Autodesk Inventor part; units mm, degrees
(part 3 of 4)
sketch "Sketch8" plane through (0, 0, 0) normal (0, -1, 0) x (1, 0, 0)
  line L0 (70.4026, -76.6897) -> (69.4026, -74.9577) projected
  line L1 (69.4026, -74.9577) -> (70.4026, -73.2256) projected
  line L2 (70.4026, -73.2256) -> (72.4026, -73.2256) projected
  line L3 (72.4026, -73.2256) -> (73.4026, -74.9577) projected
  line L4 (73.4026, -74.9577) -> (72.4026, -76.6897) projected
  line L5 (72.4026, -76.6897) -> (70.4026, -76.6897) projected
  line L6 (60.9385, -76.6897) -> (59.9385, -74.9577) projected
  line L7 (59.9385, -74.9577) -> (60.9385, -73.2256) projected
  line L8 (60.9385, -73.2256) -> (62.9385, -73.2256) projected
  line L9 (62.9385, -73.2256) -> (63.9385, -74.9577) projected
  line L10 (63.9385, -74.9577) -> (62.9385, -76.6897) projected
  line L11 (62.9385, -76.6897) -> (60.9385, -76.6897) projected
  line L12 (51.4744, -76.6897) -> (50.4744, -74.9577) projected
  line L13 (50.4744, -74.9577) -> (51.4744, -73.2256) projected
  line L14 (51.4744, -73.2256) -> (53.4744, -73.2256) projected
  line L15 (53.4744, -73.2256) -> (54.4744, -74.9577) projected
  line L16 (54.4744, -74.9577) -> (53.4744, -76.6897) projected
  line L17 (53.4744, -76.6897) -> (51.4744, -76.6897) projected
  line L18 (42.0103, -76.6897) -> (41.0103, -74.9577) projected
  line L19 (41.0103, -74.9577) -> (42.0103, -73.2256) projected
  line L20 (42.0103, -73.2256) -> (44.0103, -73.2256) projected
  line L21 (44.0103, -73.2256) -> (45.0103, -74.9577) projected
  line L22 (45.0103, -74.9577) -> (44.0103, -76.6897) projected
  line L23 (44.0103, -76.6897) -> (42.0103, -76.6897) projected
  line L24 (32.5462, -76.6897) -> (31.5462, -74.9577) projected
  line L25 (31.5462, -74.9577) -> (32.5462, -73.2256) projected
  line L26 (32.5462, -73.2256) -> (34.5462, -73.2256) projected
  line L27 (34.5462, -73.2256) -> (35.5462, -74.9577) projected
  line L28 (35.5462, -74.9577) -> (34.5462, -76.6897) projected
  line L29 (34.5462, -76.6897) -> (32.5462, -76.6897) projected
  line L30 (23.0821, -76.6897) -> (22.0821, -74.9577) projected
  line L31 (22.0821, -74.9577) -> (23.0821, -73.2256) projected
  line L32 (23.0821, -73.2256) -> (25.0821, -73.2256) projected
  line L33 (25.0821, -73.2256) -> (26.0821, -74.9577) projected
  line L34 (26.0821, -74.9577) -> (25.0821, -76.6897) projected
  line L35 (25.0821, -76.6897) -> (23.0821, -76.6897) projected
  line L36 (75.1346, -73.9577) -> (74.1346, -72.2256) projected
  line L37 (74.1346, -72.2256) -> (75.1346, -70.4936) projected
  line L38 (75.1346, -70.4936) -> (77.1346, -70.4936) projected
  line L39 (77.1346, -70.4936) -> (78.1346, -72.2256) projected
  line L40 (78.1346, -72.2256) -> (77.1346, -73.9577) projected
  line L41 (77.1346, -73.9577) -> (75.1346, -73.9577) projected
  line L42 (70.4026, -71.2256) -> (69.4026, -69.4936) projected
  line L43 (69.4026, -69.4936) -> (70.4026, -67.7615) projected
  line L44 (70.4026, -67.7615) -> (72.4026, -67.7615) projected
  line L45 (72.4026, -67.7615) -> (73.4026, -69.4936) projected
  line L46 (73.4026, -69.4936) -> (72.4026, -71.2256) projected
  line L47 (72.4026, -71.2256) -> (70.4026, -71.2256) projected
  line L48 (65.6705, -73.9577) -> (64.6705, -72.2256) projected
  line L49 (64.6705, -72.2256) -> (65.6705, -70.4936) projected
  line L50 (65.6705, -70.4936) -> (67.6705, -70.4936) projected
  line L51 (67.6705, -70.4936) -> (68.6705, -72.2256) projected
  line L52 (68.6705, -72.2256) -> (67.6705, -73.9577) projected
  line L53 (67.6705, -73.9577) -> (65.6705, -73.9577) projected
  line L54 (60.9385, -71.2256) -> (59.9385, -69.4936) projected
  line L55 (59.9385, -69.4936) -> (60.9385, -67.7615) projected
  line L56 (60.9385, -67.7615) -> (62.9385, -67.7615) projected
  line L57 (62.9385, -67.7615) -> (63.9385, -69.4936) projected
  line L58 (63.9385, -69.4936) -> (62.9385, -71.2256) projected
  line L59 (62.9385, -71.2256) -> (60.9385, -71.2256) projected
  line L60 (56.2064, -73.9577) -> (55.2064, -72.2256) projected
  line L61 (55.2064, -72.2256) -> (56.2064, -70.4936) projected
  line L62 (56.2064, -70.4936) -> (58.2064, -70.4936) projected
  line L63 (58.2064, -70.4936) -> (59.2064, -72.2256) projected
  line L64 (59.2064, -72.2256) -> (58.2064, -73.9577) projected
  line L65 (58.2064, -73.9577) -> (56.2064, -73.9577) projected
  line L66 (51.4744, -71.2256) -> (50.4744, -69.4936) projected
  line L67 (50.4744, -69.4936) -> (51.4744, -67.7615) projected
  line L68 (51.4744, -67.7615) -> (53.4744, -67.7615) projected
  line L69 (53.4744, -67.7615) -> (54.4744, -69.4936) projected
  line L70 (54.4744, -69.4936) -> (53.4744, -71.2256) projected
  line L71 (53.4744, -71.2256) -> (51.4744, -71.2256) projected
  line L72 (46.7423, -73.9577) -> (45.7423, -72.2256) projected
  line L73 (45.7423, -72.2256) -> (46.7423, -70.4936) projected
  line L74 (46.7423, -70.4936) -> (48.7423, -70.4936) projected
  line L75 (48.7423, -70.4936) -> (49.7423, -72.2256) projected
  line L76 (49.7423, -72.2256) -> (48.7423, -73.9577) projected
  line L77 (48.7423, -73.9577) -> (46.7423, -73.9577) projected
  line L78 (42.0103, -71.2256) -> (41.0103, -69.4936) projected
  line L79 (41.0103, -69.4936) -> (42.0103, -67.7615) projected
  line L80 (42.0103, -67.7615) -> (44.0103, -67.7615) projected
  line L81 (44.0103, -67.7615) -> (45.0103, -69.4936) projected
  line L82 (45.0103, -69.4936) -> (44.0103, -71.2256) projected
  line L83 (44.0103, -71.2256) -> (42.0103, -71.2256) projected
  line L84 (37.2782, -73.9577) -> (36.2782, -72.2256) projected
  line L85 (36.2782, -72.2256) -> (37.2782, -70.4936) projected
  line L86 (37.2782, -70.4936) -> (39.2782, -70.4936) projected
  line L87 (39.2782, -70.4936) -> (40.2782, -72.2256) projected
  line L88 (40.2782, -72.2256) -> (39.2782, -73.9577) projected
  line L89 (39.2782, -73.9577) -> (37.2782, -73.9577) projected
  line L90 (32.5462, -71.2256) -> (31.5462, -69.4936) projected
  line L91 (31.5462, -69.4936) -> (32.5462, -67.7615) projected
  line L92 (32.5462, -67.7615) -> (34.5462, -67.7615) projected
  line L93 (34.5462, -67.7615) -> (35.5462, -69.4936) projected
  line L94 (35.5462, -69.4936) -> (34.5462, -71.2256) projected
  line L95 (34.5462, -71.2256) -> (32.5462, -71.2256) projected
  line L96 (27.8141, -73.9577) -> (26.8141, -72.2256) projected
  line L97 (26.8141, -72.2256) -> (27.8141, -70.4936) projected
  line L98 (27.8141, -70.4936) -> (29.8141, -70.4936) projected
  line L99 (29.8141, -70.4936) -> (30.8141, -72.2256) projected
  line L100 (30.8141, -72.2256) -> (29.8141, -73.9577) projected
  line L101 (29.8141, -73.9577) -> (27.8141, -73.9577) projected
  line L102 (23.0821, -71.2256) -> (22.0821, -69.4936) projected
  line L103 (22.0821, -69.4936) -> (23.0821, -67.7615) projected
  line L104 (23.0821, -67.7615) -> (25.0821, -67.7615) projected
  line L105 (25.0821, -67.7615) -> (26.0821, -69.4936) projected
  line L106 (26.0821, -69.4936) -> (25.0821, -71.2256) projected
  line L107 (25.0821, -71.2256) -> (23.0821, -71.2256) projected
  line L108 (75.1346, -68.4936) -> (74.1346, -66.7615) projected
  line L109 (74.1346, -66.7615) -> (75.1346, -65.0295) projected
  line L110 (75.1346, -65.0295) -> (77.1346, -65.0295) projected
  line L111 (77.1346, -65.0295) -> (78.1346, -66.7615) projected
  line L112 (78.1346, -66.7615) -> (77.1346, -68.4936) projected
  line L113 (77.1346, -68.4936) -> (75.1346, -68.4936) projected
  line L114 (70.4026, -65.7615) -> (69.4026, -64.0295) projected
  line L115 (69.4026, -64.0295) -> (70.4026, -62.2974) projected
  line L116 (70.4026, -62.2974) -> (72.4026, -62.2974) projected
  line L117 (72.4026, -62.2974) -> (73.4026, -64.0295) projected
  line L118 (73.4026, -64.0295) -> (72.4026, -65.7615) projected
  line L119 (72.4026, -65.7615) -> (70.4026, -65.7615) projected
  line L120 (65.6705, -68.4936) -> (64.6705, -66.7615) projected
  line L121 (64.6705, -66.7615) -> (65.6705, -65.0295) projected
  line L122 (65.6705, -65.0295) -> (67.6705, -65.0295) projected
  line L123 (67.6705, -65.0295) -> (68.6705, -66.7615) projected
  line L124 (68.6705, -66.7615) -> (67.6705, -68.4936) projected
  line L125 (67.6705, -68.4936) -> (65.6705, -68.4936) projected
  line L126 (60.9385, -65.7615) -> (59.9385, -64.0295) projected
  line L127 (59.9385, -64.0295) -> (60.9385, -62.2974) projected
  line L128 (60.9385, -62.2974) -> (62.9385, -62.2974) projected
  line L129 (62.9385, -62.2974) -> (63.9385, -64.0295) projected
  line L130 (63.9385, -64.0295) -> (62.9385, -65.7615) projected
  line L131 (62.9385, -65.7615) -> (60.9385, -65.7615) projected
  line L132 (56.2064, -68.4936) -> (55.2064, -66.7615) projected
  line L133 (55.2064, -66.7615) -> (56.2064, -65.0295) projected
  line L134 (56.2064, -65.0295) -> (58.2064, -65.0295) projected
  line L135 (58.2064, -65.0295) -> (59.2064, -66.7615) projected
  line L136 (59.2064, -66.7615) -> (58.2064, -68.4936) projected
  line L137 (58.2064, -68.4936) -> (56.2064, -68.4936) projected
  line L138 (51.4744, -65.7615) -> (50.4744, -64.0295) projected
  line L139 (50.4744, -64.0295) -> (51.4744, -62.2974) projected
  line L140 (51.4744, -62.2974) -> (53.4744, -62.2974) projected
  line L141 (53.4744, -62.2974) -> (54.4744, -64.0295) projected
  line L142 (54.4744, -64.0295) -> (53.4744, -65.7615) projected
  line L143 (53.4744, -65.7615) -> (51.4744, -65.7615) projected
  line L144 (46.7423, -68.4936) -> (45.7423, -66.7615) projected
  line L145 (45.7423, -66.7615) -> (46.7423, -65.0295) projected
  line L146 (46.7423, -65.0295) -> (48.7423, -65.0295) projected
  line L147 (48.7423, -65.0295) -> (49.7423, -66.7615) projected
  line L148 (49.7423, -66.7615) -> (48.7423, -68.4936) projected
  line L149 (48.7423, -68.4936) -> (46.7423, -68.4936) projected
  line L150 (42.0103, -65.7615) -> (41.0103, -64.0295) projected
  line L151 (41.0103, -64.0295) -> (42.0103, -62.2974) projected
  line L152 (42.0103, -62.2974) -> (44.0103, -62.2974) projected
  line L153 (44.0103, -62.2974) -> (45.0103, -64.0295) projected
  line L154 (45.0103, -64.0295) -> (44.0103, -65.7615) projected
  line L155 (44.0103, -65.7615) -> (42.0103, -65.7615) projected
  line L156 (37.2782, -68.4936) -> (36.2782, -66.7615) projected
  line L157 (36.2782, -66.7615) -> (37.2782, -65.0295) projected
  line L158 (37.2782, -65.0295) -> (39.2782, -65.0295) projected
  line L159 (39.2782, -65.0295) -> (40.2782, -66.7615) projected
  line L160 (40.2782, -66.7615) -> (39.2782, -68.4936) projected
  line L161 (39.2782, -68.4936) -> (37.2782, -68.4936) projected
  line L162 (32.5462, -65.7615) -> (31.5462, -64.0295) projected
  line L163 (31.5462, -64.0295) -> (32.5462, -62.2974) projected
  line L164 (32.5462, -62.2974) -> (34.5462, -62.2974) projected
  line L165 (34.5462, -62.2974) -> (35.5462, -64.0295) projected
  line L166 (35.5462, -64.0295) -> (34.5462, -65.7615) projected
  line L167 (34.5462, -65.7615) -> (32.5462, -65.7615) projected
  line L168 (27.8141, -68.4936) -> (26.8141, -66.7615) projected
  line L169 (26.8141, -66.7615) -> (27.8141, -65.0295) projected
  line L170 (27.8141, -65.0295) -> (29.8141, -65.0295) projected
  line L171 (29.8141, -65.0295) -> (30.8141, -66.7615) projected
  line L172 (30.8141, -66.7615) -> (29.8141, -68.4936) projected
  line L173 (29.8141, -68.4936) -> (27.8141, -68.4936) projected
  line L174 (23.0821, -65.7615) -> (22.0821, -64.0295) projected
  line L175 (22.0821, -64.0295) -> (23.0821, -62.2974) projected
  line L176 (23.0821, -62.2974) -> (25.0821, -62.2974) projected
  line L177 (25.0821, -62.2974) -> (26.0821, -64.0295) projected
  line L178 (26.0821, -64.0295) -> (25.0821, -65.7615) projected
  line L179 (25.0821, -65.7615) -> (23.0821, -65.7615) projected
  line L180 (75.1346, -63.0295) -> (74.1346, -61.2974) projected
  line L181 (74.1346, -61.2974) -> (75.1346, -59.5654) projected
  line L182 (75.1346, -59.5654) -> (77.1346, -59.5654) projected
  line L183 (77.1346, -59.5654) -> (78.1346, -61.2974) projected
  line L184 (78.1346, -61.2974) -> (77.1346, -63.0295) projected
  line L185 (77.1346, -63.0295) -> (75.1346, -63.0295) projected
  line L186 (70.4026, -60.2974) -> (69.4026, -58.5654) projected
  line L187 (69.4026, -58.5654) -> (70.4026, -56.8333) projected
  line L188 (70.4026, -56.8333) -> (72.4026, -56.8333) projected
  line L189 (72.4026, -56.8333) -> (73.4026, -58.5654) projected
  line L190 (73.4026, -58.5654) -> (72.4026, -60.2974) projected
  line L191 (72.4026, -60.2974) -> (70.4026, -60.2974) projected
  line L192 (65.6705, -63.0295) -> (64.6705, -61.2974) projected
  line L193 (64.6705, -61.2974) -> (65.6705, -59.5654) projected
  line L194 (65.6705, -59.5654) -> (67.6705, -59.5654) projected
  line L195 (67.6705, -59.5654) -> (68.6705, -61.2974) projected
  line L196 (68.6705, -61.2974) -> (67.6705, -63.0295) projected
  line L197 (67.6705, -63.0295) -> (65.6705, -63.0295) projected
  line L198 (60.9385, -60.2974) -> (59.9385, -58.5654) projected
  line L199 (59.9385, -58.5654) -> (60.9385, -56.8333) projected
  line L200 (60.9385, -56.8333) -> (62.9385, -56.8333) projected
  line L201 (62.9385, -56.8333) -> (63.9385, -58.5654) projected
  line L202 (63.9385, -58.5654) -> (62.9385, -60.2974) projected
  line L203 (62.9385, -60.2974) -> (60.9385, -60.2974) projected
  line L204 (56.2064, -63.0295) -> (55.2064, -61.2974) projected
  line L205 (55.2064, -61.2974) -> (56.2064, -59.5654) projected
  line L206 (56.2064, -59.5654) -> (58.2064, -59.5654) projected
  line L207 (58.2064, -59.5654) -> (59.2064, -61.2974) projected
  line L208 (59.2064, -61.2974) -> (58.2064, -63.0295) projected
  line L209 (58.2064, -63.0295) -> (56.2064, -63.0295) projected
  line L210 (51.4744, -60.2974) -> (50.4744, -58.5654) projected
  line L211 (50.4744, -58.5654) -> (51.4744, -56.8333) projected
  line L212 (51.4744, -56.8333) -> (53.4744, -56.8333) projected
  line L213 (53.4744, -56.8333) -> (54.4744, -58.5654) projected
  line L214 (54.4744, -58.5654) -> (53.4744, -60.2974) projected
  line L215 (53.4744, -60.2974) -> (51.4744, -60.2974) projected
  line L216 (46.7423, -63.0295) -> (45.7423, -61.2974) projected
  line L217 (45.7423, -61.2974) -> (46.7423, -59.5654) projected
  line L218 (46.7423, -59.5654) -> (48.7423, -59.5654) projected
  line L219 (48.7423, -59.5654) -> (49.7423, -61.2974) projected
  line L220 (49.7423, -61.2974) -> (48.7423, -63.0295) projected
  line L221 (48.7423, -63.0295) -> (46.7423, -63.0295) projected
  line L222 (42.0103, -60.2974) -> (41.0103, -58.5654) projected
  line L223 (41.0103, -58.5654) -> (42.0103, -56.8333) projected
  line L224 (42.0103, -56.8333) -> (44.0103, -56.8333) projected
  line L225 (44.0103, -56.8333) -> (45.0103, -58.5654) projected
  line L226 (45.0103, -58.5654) -> (44.0103, -60.2974) projected
  line L227 (44.0103, -60.2974) -> (42.0103, -60.2974) projected
  line L228 (37.2782, -63.0295) -> (36.2782, -61.2974) projected
  line L229 (36.2782, -61.2974) -> (37.2782, -59.5654) projected
  line L230 (37.2782, -59.5654) -> (39.2782, -59.5654) projected
  line L231 (39.2782, -59.5654) -> (40.2782, -61.2974) projected
  line L232 (40.2782, -61.2974) -> (39.2782, -63.0295) projected
  line L233 (39.2782, -63.0295) -> (37.2782, -63.0295) projected
  line L234 (32.5462, -60.2974) -> (31.5462, -58.5654) projected
  line L235 (31.5462, -58.5654) -> (32.5462, -56.8333) projected
  line L236 (32.5462, -56.8333) -> (34.5462, -56.8333) projected
  line L237 (34.5462, -56.8333) -> (35.5462, -58.5654) projected
  line L238 (35.5462, -58.5654) -> (34.5462, -60.2974) projected
  line L239 (34.5462, -60.2974) -> (32.5462, -60.2974) projected
  line L240 (27.8141, -63.0295) -> (26.8141, -61.2974) projected
  line L241 (26.8141, -61.2974) -> (27.8141, -59.5654) projected
  line L242 (27.8141, -59.5654) -> (29.8141, -59.5654) projected
  line L243 (29.8141, -59.5654) -> (30.8141, -61.2974) projected
  line L244 (30.8141, -61.2974) -> (29.8141, -63.0295) projected
  line L245 (29.8141, -63.0295) -> (27.8141, -63.0295) projected
  line L246 (23.0821, -60.2974) -> (22.0821, -58.5654) projected
  line L247 (22.0821, -58.5654) -> (23.0821, -56.8333) projected
  line L248 (23.0821, -56.8333) -> (25.0821, -56.8333) projected
  line L249 (25.0821, -56.8333) -> (26.0821, -58.5654) projected
  line L250 (26.0821, -58.5654) -> (25.0821, -60.2974) projected
  line L251 (25.0821, -60.2974) -> (23.0821, -60.2974) projected
  line L252 (75.1346, -57.5654) -> (74.1346, -55.8333) projected
  line L253 (74.1346, -55.8333) -> (75.1346, -54.1013) projected
  line L254 (75.1346, -54.1013) -> (77.1346, -54.1013) projected
  line L255 (77.1346, -54.1013) -> (78.1346, -55.8333) projected
  line L256 (78.1346, -55.8333) -> (77.1346, -57.5654) projected
  line L257 (77.1346, -57.5654) -> (75.1346, -57.5654) projected
  line L258 (70.4026, -54.8333) -> (69.4026, -53.1013) projected
  line L259 (69.4026, -53.1013) -> (70.4026, -51.3692) projected
  line L260 (70.4026, -51.3692) -> (72.4026, -51.3692) projected
  line L261 (72.4026, -51.3692) -> (73.4026, -53.1013) projected
  line L262 (73.4026, -53.1013) -> (72.4026, -54.8333) projected
  line L263 (72.4026, -54.8333) -> (70.4026, -54.8333) projected
  line L264 (65.6705, -57.5654) -> (64.6705, -55.8333) projected
  line L265 (64.6705, -55.8333) -> (65.6705, -54.1013) projected
  line L266 (65.6705, -54.1013) -> (67.6705, -54.1013) projected
  line L267 (67.6705, -54.1013) -> (68.6705, -55.8333) projected
  line L268 (68.6705, -55.8333) -> (67.6705, -57.5654) projected
  line L269 (67.6705, -57.5654) -> (65.6705, -57.5654) projected
  line L270 (60.9385, -54.8333) -> (59.9385, -53.1013) projected
  line L271 (59.9385, -53.1013) -> (60.9385, -51.3692) projected
  line L272 (60.9385, -51.3692) -> (62.9385, -51.3692) projected
  line L273 (62.9385, -51.3692) -> (63.9385, -53.1013) projected
  line L274 (63.9385, -53.1013) -> (62.9385, -54.8333) projected
  line L275 (62.9385, -54.8333) -> (60.9385, -54.8333) projected
  line L276 (56.2064, -57.5654) -> (55.2064, -55.8333) projected
  line L277 (55.2064, -55.8333) -> (56.2064, -54.1013) projected
  line L278 (56.2064, -54.1013) -> (58.2064, -54.1013) projected
  line L279 (58.2064, -54.1013) -> (59.2064, -55.8333) projected
  line L280 (59.2064, -55.8333) -> (58.2064, -57.5654) projected
  line L281 (58.2064, -57.5654) -> (56.2064, -57.5654) projected
  line L282 (51.4744, -54.8333) -> (50.4744, -53.1013) projected
  line L283 (50.4744, -53.1013) -> (51.4744, -51.3692) projected
  line L284 (51.4744, -51.3692) -> (53.4744, -51.3692) projected
  line L285 (53.4744, -51.3692) -> (54.4744, -53.1013) projected
  line L286 (54.4744, -53.1013) -> (53.4744, -54.8333) projected
  line L287 (53.4744, -54.8333) -> (51.4744, -54.8333) projected
  line L288 (46.7423, -57.5654) -> (45.7423, -55.8333) projected
  line L289 (45.7423, -55.8333) -> (46.7423, -54.1013) projected
  line L290 (46.7423, -54.1013) -> (48.7423, -54.1013) projected
  line L291 (48.7423, -54.1013) -> (49.7423, -55.8333) projected
  line L292 (49.7423, -55.8333) -> (48.7423, -57.5654) projected
  line L293 (48.7423, -57.5654) -> (46.7423, -57.5654) projected
  line L294 (42.0103, -54.8333) -> (41.0103, -53.1013) projected
  line L295 (41.0103, -53.1013) -> (42.0103, -51.3692) projected
  line L296 (42.0103, -51.3692) -> (44.0103, -51.3692) projected
  line L297 (44.0103, -51.3692) -> (45.0103, -53.1013) projected
  line L298 (45.0103, -53.1013) -> (44.0103, -54.8333) projected
  line L299 (44.0103, -54.8333) -> (42.0103, -54.8333) projected
  line L300 (37.2782, -57.5654) -> (36.2782, -55.8333) projected
  line L301 (36.2782, -55.8333) -> (37.2782, -54.1013) projected
  line L302 (37.2782, -54.1013) -> (39.2782, -54.1013) projected
  line L303 (39.2782, -54.1013) -> (40.2782, -55.8333) projected
  line L304 (40.2782, -55.8333) -> (39.2782, -57.5654) projected
  line L305 (39.2782, -57.5654) -> (37.2782, -57.5654) projected
  line L306 (32.5462, -54.8333) -> (31.5462, -53.1013) projected
  line L307 (31.5462, -53.1013) -> (32.5462, -51.3692) projected
  line L308 (32.5462, -51.3692) -> (34.5462, -51.3692) projected
  line L309 (34.5462, -51.3692) -> (35.5462, -53.1013) projected
  line L310 (35.5462, -53.1013) -> (34.5462, -54.8333) projected
  line L311 (34.5462, -54.8333) -> (32.5462, -54.8333) projected
  line L312 (27.8141, -57.5654) -> (26.8141, -55.8333) projected
  line L313 (26.8141, -55.8333) -> (27.8141, -54.1013) projected
  line L314 (27.8141, -54.1013) -> (29.8141, -54.1013) projected
  line L315 (29.8141, -54.1013) -> (30.8141, -55.8333) projected
  line L316 (30.8141, -55.8333) -> (29.8141, -57.5654) projected
  line L317 (29.8141, -57.5654) -> (27.8141, -57.5654) projected
  line L318 (23.0821, -54.8333) -> (22.0821, -53.1013) projected
  line L319 (22.0821, -53.1013) -> (23.0821, -51.3692) projected
  line L320 (23.0821, -51.3692) -> (25.0821, -51.3692) projected
  line L321 (25.0821, -51.3692) -> (26.0821, -53.1013) projected
  line L322 (26.0821, -53.1013) -> (25.0821, -54.8333) projected
  line L323 (25.0821, -54.8333) -> (23.0821, -54.8333) projected
  line L324 (75.1346, -52.1013) -> (74.1346, -50.3692) projected
  line L325 (74.1346, -50.3692) -> (75.1346, -48.6372) projected
  line L326 (75.1346, -48.6372) -> (77.1346, -48.6372) projected
  line L327 (77.1346, -48.6372) -> (78.1346, -50.3692) projected
  line L328 (78.1346, -50.3692) -> (77.1346, -52.1013) projected
  line L329 (77.1346, -52.1013) -> (75.1346, -52.1013) projected
  line L330 (70.4026, -49.3692) -> (69.4026, -47.6372) projected
  line L331 (69.4026, -47.6372) -> (70.4026, -45.9051) projected
  line L332 (70.4026, -45.9051) -> (72.4026, -45.9051) projected
  line L333 (72.4026, -45.9051) -> (73.4026, -47.6372) projected
  line L334 (73.4026, -47.6372) -> (72.4026, -49.3692) projected
  line L335 (72.4026, -49.3692) -> (70.4026, -49.3692) projected
  line L336 (65.6705, -52.1013) -> (64.6705, -50.3692) projected
  line L337 (64.6705, -50.3692) -> (65.6705, -48.6372) projected
  line L338 (65.6705, -48.6372) -> (67.6705, -48.6372) projected
  line L339 (67.6705, -48.6372) -> (68.6705, -50.3692) projected
  line L340 (68.6705, -50.3692) -> (67.6705, -52.1013) projected
  line L341 (67.6705, -52.1013) -> (65.6705, -52.1013) projected
  line L342 (60.9385, -49.3692) -> (59.9385, -47.6372) projected
  line L343 (59.9385, -47.6372) -> (60.9385, -45.9051) projected
  line L344 (60.9385, -45.9051) -> (62.9385, -45.9051) projected
  line L345 (62.9385, -45.9051) -> (63.9385, -47.6372) projected
  line L346 (63.9385, -47.6372) -> (62.9385, -49.3692) projected
  line L347 (62.9385, -49.3692) -> (60.9385, -49.3692) projected
  line L348 (56.2064, -52.1013) -> (55.2064, -50.3692) projected
  line L349 (55.2064, -50.3692) -> (56.2064, -48.6372) projected
  line L350 (56.2064, -48.6372) -> (58.2064, -48.6372) projected
  line L351 (58.2064, -48.6372) -> (59.2064, -50.3692) projected
  line L352 (59.2064, -50.3692) -> (58.2064, -52.1013) projected
  line L353 (58.2064, -52.1013) -> (56.2064, -52.1013) projected
  line L354 (51.4744, -49.3692) -> (50.4744, -47.6372) projected
  line L355 (50.4744, -47.6372) -> (51.4744, -45.9051) projected
  line L356 (51.4744, -45.9051) -> (53.4744, -45.9051) projected
  line L357 (53.4744, -45.9051) -> (54.4744, -47.6372) projected
  line L358 (54.4744, -47.6372) -> (53.4744, -49.3692) projected
  line L359 (53.4744, -49.3692) -> (51.4744, -49.3692) projected
  line L360 (46.7423, -52.1013) -> (45.7423, -50.3692) projected
  line L361 (45.7423, -50.3692) -> (46.7423, -48.6372) projected
  line L362 (46.7423, -48.6372) -> (48.7423, -48.6372) projected
  line L363 (48.7423, -48.6372) -> (49.7423, -50.3692) projected
  line L364 (49.7423, -50.3692) -> (48.7423, -52.1013) projected
  line L365 (48.7423, -52.1013) -> (46.7423, -52.1013) projected
  line L366 (42.0103, -49.3692) -> (41.0103, -47.6372) projected
  line L367 (41.0103, -47.6372) -> (42.0103, -45.9051) projected
  line L368 (42.0103, -45.9051) -> (44.0103, -45.9051) projected
  line L369 (44.0103, -45.9051) -> (45.0103, -47.6372) projected
  line L370 (45.0103, -47.6372) -> (44.0103, -49.3692) projected
  line L371 (44.0103, -49.3692) -> (42.0103, -49.3692) projected
  line L372 (37.2782, -52.1013) -> (36.2782, -50.3692) projected
  line L373 (36.2782, -50.3692) -> (37.2782, -48.6372) projected
  line L374 (37.2782, -48.6372) -> (39.2782, -48.6372) projected
  line L375 (39.2782, -48.6372) -> (40.2782, -50.3692) projected
  line L376 (40.2782, -50.3692) -> (39.2782, -52.1013) projected
  line L377 (39.2782, -52.1013) -> (37.2782, -52.1013) projected
  line L378 (32.5462, -49.3692) -> (31.5462, -47.6372) projected
  line L379 (31.5462, -47.6372) -> (32.5462, -45.9051) projected
  line L380 (32.5462, -45.9051) -> (34.5462, -45.9051) projected
  line L381 (34.5462, -45.9051) -> (35.5462, -47.6372) projected
  line L382 (35.5462, -47.6372) -> (34.5462, -49.3692) projected
  line L383 (34.5462, -49.3692) -> (32.5462, -49.3692) projected
  line L384 (27.8141, -52.1013) -> (26.8141, -50.3692) projected
  line L385 (26.8141, -50.3692) -> (27.8141, -48.6372) projected
  line L386 (27.8141, -48.6372) -> (29.8141, -48.6372) projected
  line L387 (29.8141, -48.6372) -> (30.8141, -50.3692) projected
  line L388 (30.8141, -50.3692) -> (29.8141, -52.1013) projected
  line L389 (29.8141, -52.1013) -> (27.8141, -52.1013) projected
  line L390 (23.0821, -49.3692) -> (22.0821, -47.6372) projected
  line L391 (22.0821, -47.6372) -> (23.0821, -45.9051) projected
  line L392 (23.0821, -45.9051) -> (25.0821, -45.9051) projected
  line L393 (25.0821, -45.9051) -> (26.0821, -47.6372) projected
  line L394 (26.0821, -47.6372) -> (25.0821, -49.3692) projected
  line L395 (25.0821, -49.3692) -> (23.0821, -49.3692) projected
  line L396 (75.1346, -46.6372) -> (74.1346, -44.9051) projected
  line L397 (74.1346, -44.9051) -> (75.1346, -43.1731) projected
  line L398 (75.1346, -43.1731) -> (77.1346, -43.1731) projected
  line L399 (77.1346, -43.1731) -> (78.1346, -44.9051) projected
  line L400 (78.1346, -44.9051) -> (77.1346, -46.6372) projected
  line L401 (77.1346, -46.6372) -> (75.1346, -46.6372) projected
  line L402 (70.4026, -43.9051) -> (69.4026, -42.1731) projected
  line L403 (69.4026, -42.1731) -> (70.4026, -40.441) projected
  line L404 (70.4026, -40.441) -> (72.4026, -40.441) projected
  line L405 (72.4026, -40.441) -> (73.4026, -42.1731) projected
  line L406 (73.4026, -42.1731) -> (72.4026, -43.9051) projected
  line L407 (72.4026, -43.9051) -> (70.4026, -43.9051) projected
  line L408 (65.6705, -46.6372) -> (64.6705, -44.9051) projected
  line L409 (64.6705, -44.9051) -> (65.6705, -43.1731) projected
  line L410 (65.6705, -43.1731) -> (67.6705, -43.1731) projected
  line L411 (67.6705, -43.1731) -> (68.6705, -44.9051) projected
  line L412 (68.6705, -44.9051) -> (67.6705, -46.6372) projected
  line L413 (67.6705, -46.6372) -> (65.6705, -46.6372) projected
  line L414 (60.9385, -43.9051) -> (59.9385, -42.1731) projected
  line L415 (59.9385, -42.1731) -> (60.9385, -40.441) projected
  line L416 (60.9385, -40.441) -> (62.9385, -40.441) projected
  line L417 (62.9385, -40.441) -> (63.9385, -42.1731) projected
  line L418 (63.9385, -42.1731) -> (62.9385, -43.9051) projected
  line L419 (62.9385, -43.9051) -> (60.9385, -43.9051) projected
  line L420 (56.2064, -46.6372) -> (55.2064, -44.9051) projected
  line L421 (55.2064, -44.9051) -> (56.2064, -43.1731) projected
  line L422 (56.2064, -43.1731) -> (58.2064, -43.1731) projected
  line L423 (58.2064, -43.1731) -> (59.2064, -44.9051) projected
  line L424 (59.2064, -44.9051) -> (58.2064, -46.6372) projected
  line L425 (58.2064, -46.6372) -> (56.2064, -46.6372) projected
  line L426 (51.4744, -43.9051) -> (50.4744, -42.1731) projected
  line L427 (50.4744, -42.1731) -> (51.4744, -40.441) projected
  line L428 (51.4744, -40.441) -> (53.4744, -40.441) projected
  line L429 (53.4744, -40.441) -> (54.4744, -42.1731) projected
  line L430 (54.4744, -42.1731) -> (53.4744, -43.9051) projected
  line L431 (53.4744, -43.9051) -> (51.4744, -43.9051) projected
  line L432 (46.7423, -46.6372) -> (45.7423, -44.9051) projected
  line L433 (45.7423, -44.9051) -> (46.7423, -43.1731) projected
  line L434 (46.7423, -43.1731) -> (48.7423, -43.1731) projected
  line L435 (48.7423, -43.1731) -> (49.7423, -44.9051) projected
  line L436 (49.7423, -44.9051) -> (48.7423, -46.6372) projected
  line L437 (48.7423, -46.6372) -> (46.7423, -46.6372) projected
  line L438 (42.0103, -43.9051) -> (41.0103, -42.1731) projected
  line L439 (41.0103, -42.1731) -> (42.0103, -40.441) projected
  line L440 (42.0103, -40.441) -> (44.0103, -40.441) projected
  line L441 (44.0103, -40.441) -> (45.0103, -42.1731) projected
  line L442 (45.0103, -42.1731) -> (44.0103, -43.9051) projected
  line L443 (44.0103, -43.9051) -> (42.0103, -43.9051) projected
  line L444 (37.2782, -46.6372) -> (36.2782, -44.9051) projected
  line L445 (36.2782, -44.9051) -> (37.2782, -43.1731) projected
  line L446 (37.2782, -43.1731) -> (39.2782, -43.1731) projected
  line L447 (39.2782, -43.1731) -> (40.2782, -44.9051) projected
  line L448 (40.2782, -44.9051) -> (39.2782, -46.6372) projected
  line L449 (39.2782, -46.6372) -> (37.2782, -46.6372) projected
  line L450 (32.5462, -43.9051) -> (31.5462, -42.1731) projected
  line L451 (31.5462, -42.1731) -> (32.5462, -40.441) projected
  line L452 (32.5462, -40.441) -> (34.5462, -40.441) projected
  line L453 (34.5462, -40.441) -> (35.5462, -42.1731) projected
  line L454 (35.5462, -42.1731) -> (34.5462, -43.9051) projected
  line L455 (34.5462, -43.9051) -> (32.5462, -43.9051) projected
  line L456 (27.8141, -46.6372) -> (26.8141, -44.9051) projected
  line L457 (26.8141, -44.9051) -> (27.8141, -43.1731) projected
  line L458 (27.8141, -43.1731) -> (29.8141, -43.1731) projected
  line L459 (29.8141, -43.1731) -> (30.8141, -44.9051) projected
  line L460 (30.8141, -44.9051) -> (29.8141, -46.6372) projected
  line L461 (29.8141, -46.6372) -> (27.8141, -46.6372) projected
  line L462 (23.0821, -43.9051) -> (22.0821, -42.1731) projected
  line L463 (22.0821, -42.1731) -> (23.0821, -40.441) projected
  line L464 (23.0821, -40.441) -> (25.0821, -40.441) projected
  line L465 (25.0821, -40.441) -> (26.0821, -42.1731) projected
  line L466 (26.0821, -42.1731) -> (25.0821, -43.9051) projected
  line L467 (25.0821, -43.9051) -> (23.0821, -43.9051) projected
  line L468 (75.1346, -41.1731) -> (74.1346, -39.441) projected
  line L469 (74.1346, -39.441) -> (75.1346, -37.709) projected
  line L470 (75.1346, -37.709) -> (77.1346, -37.709) projected
  line L471 (77.1346, -37.709) -> (78.1346, -39.441) projected
  line L472 (78.1346, -39.441) -> (77.1346, -41.1731) projected
  line L473 (77.1346, -41.1731) -> (75.1346, -41.1731) projected
  line L474 (70.4026, -38.441) -> (69.4026, -36.709) projected
  line L475 (69.4026, -36.709) -> (70.4026, -34.9769) projected
  line L476 (70.4026, -34.9769) -> (72.4026, -34.9769) projected
  line L477 (72.4026, -34.9769) -> (73.4026, -36.709) projected
  line L478 (73.4026, -36.709) -> (72.4026, -38.441) projected
  line L479 (72.4026, -38.441) -> (70.4026, -38.441) projected
  line L480 (65.6705, -41.1731) -> (64.6705, -39.441) projected
  line L481 (64.6705, -39.441) -> (65.6705, -37.709) projected
  line L482 (65.6705, -37.709) -> (67.6705, -37.709) projected
  line L483 (67.6705, -37.709) -> (68.6705, -39.441) projected
  line L484 (68.6705, -39.441) -> (67.6705, -41.1731) projected
  line L485 (67.6705, -41.1731) -> (65.6705, -41.1731) projected
  line L486 (60.9385, -38.441) -> (59.9385, -36.709) projected
  line L487 (59.9385, -36.709) -> (60.9385, -34.9769) projected
  line L488 (60.9385, -34.9769) -> (62.9385, -34.9769) projected
  line L489 (62.9385, -34.9769) -> (63.9385, -36.709) projected
  line L490 (63.9385, -36.709) -> (62.9385, -38.441) projected
  line L491 (62.9385, -38.441) -> (60.9385, -38.441) projected
  line L492 (56.2064, -41.1731) -> (55.2064, -39.441) projected
  line L493 (55.2064, -39.441) -> (56.2064, -37.709) projected
  line L494 (56.2064, -37.709) -> (58.2064, -37.709) projected
  line L495 (58.2064, -37.709) -> (59.2064, -39.441) projected
  line L496 (59.2064, -39.441) -> (58.2064, -41.1731) projected
  line L497 (58.2064, -41.1731) -> (56.2064, -41.1731) projected
  line L498 (51.4744, -38.441) -> (50.4744, -36.709) projected
  line L499 (50.4744, -36.709) -> (51.4744, -34.9769) projected
  line L500 (51.4744, -34.9769) -> (53.4744, -34.9769) projected
  line L501 (53.4744, -34.9769) -> (54.4744, -36.709) projected
  line L502 (54.4744, -36.709) -> (53.4744, -38.441) projected
  line L503 (53.4744, -38.441) -> (51.4744, -38.441) projected
  line L504 (46.7423, -41.1731) -> (45.7423, -39.441) projected
  line L505 (45.7423, -39.441) -> (46.7423, -37.709) projected
  line L506 (46.7423, -37.709) -> (48.7423, -37.709) projected
  line L507 (48.7423, -37.709) -> (49.7423, -39.441) projected
  line L508 (49.7423, -39.441) -> (48.7423, -41.1731) projected
  line L509 (48.7423, -41.1731) -> (46.7423, -41.1731) projected
  line L510 (42.0103, -38.441) -> (41.0103, -36.709) projected
  line L511 (41.0103, -36.709) -> (42.0103, -34.9769) projected
  line L512 (42.0103, -34.9769) -> (44.0103, -34.9769) projected
  line L513 (44.0103, -34.9769) -> (45.0103, -36.709) projected
  line L514 (45.0103, -36.709) -> (44.0103, -38.441) projected
  line L515 (44.0103, -38.441) -> (42.0103, -38.441) projected
  line L516 (37.2782, -41.1731) -> (36.2782, -39.441) projected
  line L517 (36.2782, -39.441) -> (37.2782, -37.709) projected
  line L518 (37.2782, -37.709) -> (39.2782, -37.709) projected
  line L519 (39.2782, -37.709) -> (40.2782, -39.441) projected
  line L520 (40.2782, -39.441) -> (39.2782, -41.1731) projected
  line L521 (39.2782, -41.1731) -> (37.2782, -41.1731) projected
  line L522 (32.5462, -38.441) -> (31.5462, -36.709) projected
  line L523 (31.5462, -36.709) -> (32.5462, -34.9769) projected
  line L524 (32.5462, -34.9769) -> (34.5462, -34.9769) projected
  line L525 (34.5462, -34.9769) -> (35.5462, -36.709) projected
  line L526 (35.5462, -36.709) -> (34.5462, -38.441) projected
  line L527 (34.5462, -38.441) -> (32.5462, -38.441) projected
  line L528 (27.8141, -41.1731) -> (26.8141, -39.441) projected
  line L529 (26.8141, -39.441) -> (27.8141, -37.709) projected
  line L530 (27.8141, -37.709) -> (29.8141, -37.709) projected
  line L531 (29.8141, -37.709) -> (30.8141, -39.441) projected
  line L532 (30.8141, -39.441) -> (29.8141, -41.1731) projected
  line L533 (29.8141, -41.1731) -> (27.8141, -41.1731) projected
  line L534 (23.0821, -38.441) -> (22.0821, -36.709) projected
  line L535 (22.0821, -36.709) -> (23.0821, -34.9769) projected
  line L536 (23.0821, -34.9769) -> (25.0821, -34.9769) projected
  line L537 (25.0821, -34.9769) -> (26.0821, -36.709) projected
  line L538 (26.0821, -36.709) -> (25.0821, -38.441) projected
  line L539 (25.0821, -38.441) -> (23.0821, -38.441) projected
  line L540 (75.1346, -35.709) -> (74.1346, -33.9769) projected
  line L541 (74.1346, -33.9769) -> (75.1346, -32.2449) projected
  line L542 (75.1346, -32.2449) -> (77.1346, -32.2449) projected
  line L543 (77.1346, -32.2449) -> (78.1346, -33.9769) projected
  line L544 (78.1346, -33.9769) -> (77.1346, -35.709) projected
  line L545 (77.1346, -35.709) -> (75.1346, -35.709) projected
  line L546 (70.4026, -32.9769) -> (69.4026, -31.2449) projected
  line L547 (69.4026, -31.2449) -> (70.4026, -29.5128) projected
  line L548 (70.4026, -29.5128) -> (72.4026, -29.5128) projected
  line L549 (72.4026, -29.5128) -> (73.4026, -31.2449) projected
  line L550 (73.4026, -31.2449) -> (72.4026, -32.9769) projected
  line L551 (72.4026, -32.9769) -> (70.4026, -32.9769) projected
  line L552 (65.6705, -35.709) -> (64.6705, -33.9769) projected
  line L553 (64.6705, -33.9769) -> (65.6705, -32.2449) projected
  line L554 (65.6705, -32.2449) -> (67.6705, -32.2449) projected
  line L555 (67.6705, -32.2449) -> (68.6705, -33.9769) projected
  line L556 (68.6705, -33.9769) -> (67.6705, -35.709) projected
  line L557 (67.6705, -35.709) -> (65.6705, -35.709) projected
  line L558 (60.9385, -32.9769) -> (59.9385, -31.2449) projected
  line L559 (59.9385, -31.2449) -> (60.9385, -29.5128) projected
  line L560 (60.9385, -29.5128) -> (62.9385, -29.5128) projected
  line L561 (62.9385, -29.5128) -> (63.9385, -31.2449) projected
  line L562 (63.9385, -31.2449) -> (62.9385, -32.9769) projected
  line L563 (62.9385, -32.9769) -> (60.9385, -32.9769) projected
  line L564 (56.2064, -35.709) -> (55.2064, -33.9769) projected
  line L565 (55.2064, -33.9769) -> (56.2064, -32.2449) projected
  line L566 (56.2064, -32.2449) -> (58.2064, -32.2449) projected
  line L567 (58.2064, -32.2449) -> (59.2064, -33.9769) projected
  line L568 (59.2064, -33.9769) -> (58.2064, -35.709) projected
  line L569 (58.2064, -35.709) -> (56.2064, -35.709) projected
  line L570 (51.4744, -32.9769) -> (50.4744, -31.2449) projected
  line L571 (50.4744, -31.2449) -> (51.4744, -29.5128) projected
  line L572 (51.4744, -29.5128) -> (53.4744, -29.5128) projected
  line L573 (53.4744, -29.5128) -> (54.4744, -31.2449) projected
  line L574 (54.4744, -31.2449) -> (53.4744, -32.9769) projected
  line L575 (53.4744, -32.9769) -> (51.4744, -32.9769) projected
  line L576 (46.7423, -35.709) -> (45.7423, -33.9769) projected
  line L577 (45.7423, -33.9769) -> (46.7423, -32.2449) projected
  line L578 (46.7423, -32.2449) -> (48.7423, -32.2449) projected
  line L579 (48.7423, -32.2449) -> (49.7423, -33.9769) projected
  line L580 (49.7423, -33.9769) -> (48.7423, -35.709) projected
  line L581 (48.7423, -35.709) -> (46.7423, -35.709) projected
  line L582 (42.0103, -32.9769) -> (41.0103, -31.2449) projected
  line L583 (41.0103, -31.2449) -> (42.0103, -29.5128) projected
  line L584 (42.0103, -29.5128) -> (44.0103, -29.5128) projected
  line L585 (44.0103, -29.5128) -> (45.0103, -31.2449) projected
  line L586 (45.0103, -31.2449) -> (44.0103, -32.9769) projected
  line L587 (44.0103, -32.9769) -> (42.0103, -32.9769) projected
  line L588 (37.2782, -35.709) -> (36.2782, -33.9769) projected
  line L589 (36.2782, -33.9769) -> (37.2782, -32.2449) projected
  line L590 (37.2782, -32.2449) -> (39.2782, -32.2449) projected
  line L591 (39.2782, -32.2449) -> (40.2782, -33.9769) projected
  line L592 (40.2782, -33.9769) -> (39.2782, -35.709) projected
  line L593 (39.2782, -35.709) -> (37.2782, -35.709) projected
  line L594 (32.5462, -32.9769) -> (31.5462, -31.2449) projected
  line L595 (31.5462, -31.2449) -> (32.5462, -29.5128) projected
  line L596 (32.5462, -29.5128) -> (34.5462, -29.5128) projected
  line L597 (34.5462, -29.5128) -> (35.5462, -31.2449) projected
  line L598 (35.5462, -31.2449) -> (34.5462, -32.9769) projected
  line L599 (34.5462, -32.9769) -> (32.5462, -32.9769) projected
  line L600 (27.8141, -35.709) -> (26.8141, -33.9769) projected
  line L601 (26.8141, -33.9769) -> (27.8141, -32.2449) projected
  line L602 (27.8141, -32.2449) -> (29.8141, -32.2449) projected
  line L603 (29.8141, -32.2449) -> (30.8141, -33.9769) projected
  line L604 (30.8141, -33.9769) -> (29.8141, -35.709) projected
  line L605 (29.8141, -35.709) -> (27.8141, -35.709) projected
  line L606 (23.0821, -32.9769) -> (22.0821, -31.2449) projected
  line L607 (22.0821, -31.2449) -> (23.0821, -29.5128) projected
  line L608 (23.0821, -29.5128) -> (25.0821, -29.5128) projected
  line L609 (25.0821, -29.5128) -> (26.0821, -31.2449) projected
  line L610 (26.0821, -31.2449) -> (25.0821, -32.9769) projected
  line L611 (25.0821, -32.9769) -> (23.0821, -32.9769) projected
  line L612 (75.1346, -30.2449) -> (74.1346, -28.5128) projected
  line L613 (74.1346, -28.5128) -> (75.1346, -26.7808) projected
  line L614 (75.1346, -26.7808) -> (77.1346, -26.7808) projected
  line L615 (77.1346, -26.7808) -> (78.1346, -28.5128) projected
  line L616 (78.1346, -28.5128) -> (77.1346, -30.2449) projected
  line L617 (77.1346, -30.2449) -> (75.1346, -30.2449) projected
  line L618 (70.4026, -27.5128) -> (69.4026, -25.7808) projected
  line L619 (69.4026, -25.7808) -> (70.4026, -24.0487) projected
  line L620 (70.4026, -24.0487) -> (72.4026, -24.0487) projected
  line L621 (72.4026, -24.0487) -> (73.4026, -25.7808) projected
  line L622 (73.4026, -25.7808) -> (72.4026, -27.5128) projected
  line L623 (72.4026, -27.5128) -> (70.4026, -27.5128) projected
  line L624 (65.6705, -30.2449) -> (64.6705, -28.5128) projected
  line L625 (64.6705, -28.5128) -> (65.6705, -26.7808) projected
  line L626 (65.6705, -26.7808) -> (67.6705, -26.7808) projected
  line L627 (67.6705, -26.7808) -> (68.6705, -28.5128) projected
  line L628 (68.6705, -28.5128) -> (67.6705, -30.2449) projected
  line L629 (67.6705, -30.2449) -> (65.6705, -30.2449) projected
  line L630 (60.9385, -27.5128) -> (59.9385, -25.7808) projected
  line L631 (59.9385, -25.7808) -> (60.9385, -24.0487) projected
  line L632 (60.9385, -24.0487) -> (62.9385, -24.0487) projected
  line L633 (62.9385, -24.0487) -> (63.9385, -25.7808) projected
  line L634 (63.9385, -25.7808) -> (62.9385, -27.5128) projected
  line L635 (62.9385, -27.5128) -> (60.9385, -27.5128) projected
  line L636 (56.2064, -30.2449) -> (55.2064, -28.5128) projected
  line L637 (55.2064, -28.5128) -> (56.2064, -26.7808) projected
  line L638 (56.2064, -26.7808) -> (58.2064, -26.7808) projected
  line L639 (58.2064, -26.7808) -> (59.2064, -28.5128) projected
  line L640 (59.2064, -28.5128) -> (58.2064, -30.2449) projected
  line L641 (58.2064, -30.2449) -> (56.2064, -30.2449) projected
  line L642 (51.4744, -27.5128) -> (50.4744, -25.7808) projected
  line L643 (50.4744, -25.7808) -> (51.4744, -24.0487) projected
  line L644 (51.4744, -24.0487) -> (53.4744, -24.0487) projected
  line L645 (53.4744, -24.0487) -> (54.4744, -25.7808) projected
  line L646 (54.4744, -25.7808) -> (53.4744, -27.5128) projected
  line L647 (53.4744, -27.5128) -> (51.4744, -27.5128) projected
  line L648 (46.7423, -30.2449) -> (45.7423, -28.5128) projected
  line L649 (45.7423, -28.5128) -> (46.7423, -26.7808) projected
  line L650 (46.7423, -26.7808) -> (48.7423, -26.7808) projected
  line L651 (48.7423, -26.7808) -> (49.7423, -28.5128) projected
  line L652 (49.7423, -28.5128) -> (48.7423, -30.2449) projected
  line L653 (48.7423, -30.2449) -> (46.7423, -30.2449) projected
  line L654 (42.0103, -27.5128) -> (41.0103, -25.7808) projected
  line L655 (41.0103, -25.7808) -> (42.0103, -24.0487) projected
  line L656 (42.0103, -24.0487) -> (44.0103, -24.0487) projected
  line L657 (44.0103, -24.0487) -> (45.0103, -25.7808) projected
  line L658 (45.0103, -25.7808) -> (44.0103, -27.5128) projected
  line L659 (44.0103, -27.5128) -> (42.0103, -27.5128) projected
  line L660 (37.2782, -30.2449) -> (36.2782, -28.5128) projected
  line L661 (36.2782, -28.5128) -> (37.2782, -26.7808) projected
  line L662 (37.2782, -26.7808) -> (39.2782, -26.7808) projected
  line L663 (39.2782, -26.7808) -> (40.2782, -28.5128) projected
  line L664 (40.2782, -28.5128) -> (39.2782, -30.2449) projected
  line L665 (39.2782, -30.2449) -> (37.2782, -30.2449) projected
  line L666 (32.5462, -27.5128) -> (31.5462, -25.7808) projected
  line L667 (31.5462, -25.7808) -> (32.5462, -24.0487) projected
  line L668 (32.5462, -24.0487) -> (34.5462, -24.0487) projected
  line L669 (34.5462, -24.0487) -> (35.5462, -25.7808) projected
  line L670 (35.5462, -25.7808) -> (34.5462, -27.5128) projected
  line L671 (34.5462, -27.5128) -> (32.5462, -27.5128) projected
  line L672 (27.8141, -30.2449) -> (26.8141, -28.5128) projected
  line L673 (26.8141, -28.5128) -> (27.8141, -26.7808) projected
  line L674 (27.8141, -26.7808) -> (29.8141, -26.7808) projected
  line L675 (29.8141, -26.7808) -> (30.8141, -28.5128) projected
  line L676 (30.8141, -28.5128) -> (29.8141, -30.2449) projected
  line L677 (29.8141, -30.2449) -> (27.8141, -30.2449) projected
  line L678 (23.0821, -27.5128) -> (22.0821, -25.7808) projected
  line L679 (22.0821, -25.7808) -> (23.0821, -24.0487) projected
  line L680 (23.0821, -24.0487) -> (25.0821, -24.0487) projected
  line L681 (25.0821, -24.0487) -> (26.0821, -25.7808) projected
  line L682 (26.0821, -25.7808) -> (25.0821, -27.5128) projected
  line L683 (25.0821, -27.5128) -> (23.0821, -27.5128) projected
  line L684 (75.1346, -24.7808) -> (74.1346, -23.0487) projected
  line L685 (74.1346, -23.0487) -> (75.1346, -21.3167) projected
  line L686 (75.1346, -21.3167) -> (77.1346, -21.3167) projected
  line L687 (77.1346, -21.3167) -> (78.1346, -23.0487) projected
  line L688 (78.1346, -23.0487) -> (77.1346, -24.7808) projected
  line L689 (77.1346, -24.7808) -> (75.1346, -24.7808) projected
  line L690 (70.4026, -22.0487) -> (69.4026, -20.3167) projected
  line L691 (69.4026, -20.3167) -> (70.4026, -18.5846) projected
  line L692 (70.4026, -18.5846) -> (72.4026, -18.5846) projected
  line L693 (72.4026, -18.5846) -> (73.4026, -20.3167) projected
  line L694 (73.4026, -20.3167) -> (72.4026, -22.0487) projected
  line L695 (72.4026, -22.0487) -> (70.4026, -22.0487) projected
  line L696 (65.6705, -24.7808) -> (64.6705, -23.0487) projected
  line L697 (64.6705, -23.0487) -> (65.6705, -21.3167) projected
  line L698 (65.6705, -21.3167) -> (67.6705, -21.3167) projected
  line L699 (67.6705, -21.3167) -> (68.6705, -23.0487) projected
  line L700 (68.6705, -23.0487) -> (67.6705, -24.7808) projected
  line L701 (67.6705, -24.7808) -> (65.6705, -24.7808) projected
  line L702 (60.9385, -22.0487) -> (59.9385, -20.3167) projected
  line L703 (59.9385, -20.3167) -> (60.9385, -18.5846) projected
  line L704 (60.9385, -18.5846) -> (62.9385, -18.5846) projected
  line L705 (62.9385, -18.5846) -> (63.9385, -20.3167) projected
  line L706 (63.9385, -20.3167) -> (62.9385, -22.0487) projected
  line L707 (62.9385, -22.0487) -> (60.9385, -22.0487) projected
  line L708 (56.2064, -24.7808) -> (55.2064, -23.0487) projected
  line L709 (55.2064, -23.0487) -> (56.2064, -21.3167) projected
  line L710 (56.2064, -21.3167) -> (58.2064, -21.3167) projected
  line L711 (58.2064, -21.3167) -> (59.2064, -23.0487) projected
  line L712 (59.2064, -23.0487) -> (58.2064, -24.7808) projected
  line L713 (58.2064, -24.7808) -> (56.2064, -24.7808) projected
  line L714 (51.4744, -22.0487) -> (50.4744, -20.3167) projected
  line L715 (50.4744, -20.3167) -> (51.4744, -18.5846) projected
  line L716 (51.4744, -18.5846) -> (53.4744, -18.5846) projected
  line L717 (53.4744, -18.5846) -> (54.4744, -20.3167) projected
  line L718 (54.4744, -20.3167) -> (53.4744, -22.0487) projected
  line L719 (53.4744, -22.0487) -> (51.4744, -22.0487) projected
  line L720 (46.7423, -24.7808) -> (45.7423, -23.0487) projected
  line L721 (45.7423, -23.0487) -> (46.7423, -21.3167) projected
  line L722 (46.7423, -21.3167) -> (48.7423, -21.3167) projected
  line L723 (48.7423, -21.3167) -> (49.7423, -23.0487) projected
  line L724 (49.7423, -23.0487) -> (48.7423, -24.7808) projected
  line L725 (48.7423, -24.7808) -> (46.7423, -24.7808) projected
  line L726 (42.0103, -22.0487) -> (41.0103, -20.3167) projected
  line L727 (41.0103, -20.3167) -> (42.0103, -18.5846) projected
  line L728 (42.0103, -18.5846) -> (44.0103, -18.5846) projected
  line L729 (44.0103, -18.5846) -> (45.0103, -20.3167) projected
  line L730 (45.0103, -20.3167) -> (44.0103, -22.0487) projected
  line L731 (44.0103, -22.0487) -> (42.0103, -22.0487) projected
  line L732 (37.2782, -24.7808) -> (36.2782, -23.0487) projected
  line L733 (36.2782, -23.0487) -> (37.2782, -21.3167) projected
  line L734 (37.2782, -21.3167) -> (39.2782, -21.3167) projected
  line L735 (39.2782, -21.3167) -> (40.2782, -23.0487) projected
  line L736 (40.2782, -23.0487) -> (39.2782, -24.7808) projected
  line L737 (39.2782, -24.7808) -> (37.2782, -24.7808) projected
  line L738 (32.5462, -22.0487) -> (31.5462, -20.3167) projected
  line L739 (31.5462, -20.3167) -> (32.5462, -18.5846) projected
  line L740 (32.5462, -18.5846) -> (34.5462, -18.5846) projected
  line L741 (34.5462, -18.5846) -> (35.5462, -20.3167) projected
  line L742 (35.5462, -20.3167) -> (34.5462, -22.0487) projected
  line L743 (34.5462, -22.0487) -> (32.5462, -22.0487) projected
  line L744 (27.8141, -24.7808) -> (26.8141, -23.0487) projected
  line L745 (26.8141, -23.0487) -> (27.8141, -21.3167) projected
  line L746 (27.8141, -21.3167) -> (29.8141, -21.3167) projected
  line L747 (29.8141, -21.3167) -> (30.8141, -23.0487) projected
  line L748 (30.8141, -23.0487) -> (29.8141, -24.7808) projected
  line L749 (29.8141, -24.7808) -> (27.8141, -24.7808) projected
  line L750 (23.0821, -22.0487) -> (22.0821, -20.3167) projected
  line L751 (22.0821, -20.3167) -> (23.0821, -18.5846) projected
  line L752 (23.0821, -18.5846) -> (25.0821, -18.5846) projected
  line L753 (25.0821, -18.5846) -> (26.0821, -20.3167) projected
  line L754 (26.0821, -20.3167) -> (25.0821, -22.0487) projected
  line L755 (25.0821, -22.0487) -> (23.0821, -22.0487) projected
  line L756 (75.1346, -19.3167) -> (74.1346, -17.5846) projected
  line L757 (74.1346, -17.5846) -> (75.1346, -15.8526) projected
  line L758 (75.1346, -15.8526) -> (77.1346, -15.8526) projected
  line L759 (77.1346, -15.8526) -> (78.1346, -17.5846) projected
  line L760 (78.1346, -17.5846) -> (77.1346, -19.3167) projected
  line L761 (77.1346, -19.3167) -> (75.1346, -19.3167) projected
  line L762 (70.4026, -16.5846) -> (69.4026, -14.8526) projected
  line L763 (69.4026, -14.8526) -> (70.4026, -13.1205) projected
  line L764 (70.4026, -13.1205) -> (72.4026, -13.1205) projected
  line L765 (72.4026, -13.1205) -> (73.4026, -14.8526) projected
  line L766 (73.4026, -14.8526) -> (72.4026, -16.5846) projected
  line L767 (72.4026, -16.5846) -> (70.4026, -16.5846) projected
  line L768 (65.6705, -19.3167) -> (64.6705, -17.5846) projected
  line L769 (64.6705, -17.5846) -> (65.6705, -15.8526) projected
  line L770 (65.6705, -15.8526) -> (67.6705, -15.8526) projected
  line L771 (67.6705, -15.8526) -> (68.6705, -17.5846) projected
  line L772 (68.6705, -17.5846) -> (67.6705, -19.3167) projected
  line L773 (67.6705, -19.3167) -> (65.6705, -19.3167) projected
  line L774 (60.9385, -16.5846) -> (59.9385, -14.8526) projected
  line L775 (59.9385, -14.8526) -> (60.9385, -13.1205) projected
  line L776 (60.9385, -13.1205) -> (62.9385, -13.1205) projected
  line L777 (62.9385, -13.1205) -> (63.9385, -14.8526) projected
  line L778 (63.9385, -14.8526) -> (62.9385, -16.5846) projected
  line L779 (62.9385, -16.5846) -> (60.9385, -16.5846) projected
  line L780 (56.2064, -19.3167) -> (55.2064, -17.5846) projected
  line L781 (55.2064, -17.5846) -> (56.2064, -15.8526) projected
  line L782 (56.2064, -15.8526) -> (58.2064, -15.8526) projected
  line L783 (58.2064, -15.8526) -> (59.2064, -17.5846) projected
  line L784 (59.2064, -17.5846) -> (58.2064, -19.3167) projected
  line L785 (58.2064, -19.3167) -> (56.2064, -19.3167) projected
  line L786 (51.4744, -16.5846) -> (50.4744, -14.8526) projected
  line L787 (50.4744, -14.8526) -> (51.4744, -13.1205) projected
  line L788 (51.4744, -13.1205) -> (53.4744, -13.1205) projected
  line L789 (53.4744, -13.1205) -> (54.4744, -14.8526) projected
  line L790 (54.4744, -14.8526) -> (53.4744, -16.5846) projected
  line L791 (53.4744, -16.5846) -> (51.4744, -16.5846) projected
  line L792 (46.7423, -19.3167) -> (45.7423, -17.5846) projected
  line L793 (45.7423, -17.5846) -> (46.7423, -15.8526) projected
  line L794 (46.7423, -15.8526) -> (48.7423, -15.8526) projected
  line L795 (48.7423, -15.8526) -> (49.7423, -17.5846) projected
  line L796 (49.7423, -17.5846) -> (48.7423, -19.3167) projected
  line L797 (48.7423, -19.3167) -> (46.7423, -19.3167) projected
  line L798 (42.0103, -16.5846) -> (41.0103, -14.8526) projected
  line L799 (41.0103, -14.8526) -> (42.0103, -13.1205) projected
  line L800 (42.0103, -13.1205) -> (44.0103, -13.1205) projected
  line L801 (44.0103, -13.1205) -> (45.0103, -14.8526) projected
  line L802 (45.0103, -14.8526) -> (44.0103, -16.5846) projected
  line L803 (44.0103, -16.5846) -> (42.0103, -16.5846) projected
  line L804 (37.2782, -19.3167) -> (36.2782, -17.5846) projected
  line L805 (36.2782, -17.5846) -> (37.2782, -15.8526) projected
  line L806 (37.2782, -15.8526) -> (39.2782, -15.8526) projected
  line L807 (39.2782, -15.8526) -> (40.2782, -17.5846) projected
  line L808 (40.2782, -17.5846) -> (39.2782, -19.3167) projected
  line L809 (39.2782, -19.3167) -> (37.2782, -19.3167) projected
  line L810 (32.5462, -16.5846) -> (31.5462, -14.8526) projected
  line L811 (31.5462, -14.8526) -> (32.5462, -13.1205) projected
  line L812 (32.5462, -13.1205) -> (34.5462, -13.1205) projected
  line L813 (34.5462, -13.1205) -> (35.5462, -14.8526) projected
  line L814 (35.5462, -14.8526) -> (34.5462, -16.5846) projected
  line L815 (34.5462, -16.5846) -> (32.5462, -16.5846) projected
  line L816 (27.8141, -19.3167) -> (26.8141, -17.5846) projected
  line L817 (26.8141, -17.5846) -> (27.8141, -15.8526) projected
  line L818 (27.8141, -15.8526) -> (29.8141, -15.8526) projected
  line L819 (29.8141, -15.8526) -> (30.8141, -17.5846) projected
  line L820 (30.8141, -17.5846) -> (29.8141, -19.3167) projected
  line L821 (29.8141, -19.3167) -> (27.8141, -19.3167) projected
  line L822 (23.0821, -16.5846) -> (22.0821, -14.8526) projected
  line L823 (22.0821, -14.8526) -> (23.0821, -13.1205) projected
  line L824 (23.0821, -13.1205) -> (25.0821, -13.1205) projected
  line L825 (25.0821, -13.1205) -> (26.0821, -14.8526) projected
  line L826 (26.0821, -14.8526) -> (25.0821, -16.5846) projected
  line L827 (25.0821, -16.5846) -> (23.0821, -16.5846) projected
  line L828 (75.1346, -13.8526) -> (74.1346, -12.1205) projected
  line L829 (74.1346, -12.1205) -> (75.1346, -10.3885) projected
  line L830 (75.1346, -10.3885) -> (77.1346, -10.3885) projected
  line L831 (77.1346, -10.3885) -> (78.1346, -12.1205) projected
  line L832 (78.1346, -12.1205) -> (77.1346, -13.8526) projected
  line L833 (77.1346, -13.8526) -> (75.1346, -13.8526) projected
  line L834 (70.4026, -11.1205) -> (69.4026, -9.3885) projected
  line L835 (69.4026, -9.3885) -> (70.4026, -7.6564) projected
  line L836 (70.4026, -7.6564) -> (72.4026, -7.6564) projected
  line L837 (72.4026, -7.6564) -> (73.4026, -9.3885) projected
  line L838 (73.4026, -9.3885) -> (72.4026, -11.1205) projected
  line L839 (72.4026, -11.1205) -> (70.4026, -11.1205) projected
  line L840 (65.6705, -13.8526) -> (64.6705, -12.1205) projected
  line L841 (64.6705, -12.1205) -> (65.6705, -10.3885) projected
  line L842 (65.6705, -10.3885) -> (67.6705, -10.3885) projected
  line L843 (67.6705, -10.3885) -> (68.6705, -12.1205) projected
  line L844 (68.6705, -12.1205) -> (67.6705, -13.8526) projected
  line L845 (67.6705, -13.8526) -> (65.6705, -13.8526) projected
  line L846 (60.9385, -11.1205) -> (59.9385, -9.3885) projected
  line L847 (59.9385, -9.3885) -> (60.9385, -7.6564) projected
  line L848 (60.9385, -7.6564) -> (62.9385, -7.6564) projected
  line L849 (62.9385, -7.6564) -> (63.9385, -9.3885) projected
  line L850 (63.9385, -9.3885) -> (62.9385, -11.1205) projected
  line L851 (62.9385, -11.1205) -> (60.9385, -11.1205) projected
  line L852 (56.2064, -13.8526) -> (55.2064, -12.1205) projected
  line L853 (55.2064, -12.1205) -> (56.2064, -10.3885) projected
  line L854 (56.2064, -10.3885) -> (58.2064, -10.3885) projected
  line L855 (58.2064, -10.3885) -> (59.2064, -12.1205) projected
  line L856 (59.2064, -12.1205) -> (58.2064, -13.8526) projected
  line L857 (58.2064, -13.8526) -> (56.2064, -13.8526) projected
  line L858 (51.4744, -11.1205) -> (50.4744, -9.3885) projected
  line L859 (50.4744, -9.3885) -> (51.4744, -7.6564) projected
  line L860 (51.4744, -7.6564) -> (53.4744, -7.6564) projected
  line L861 (53.4744, -7.6564) -> (54.4744, -9.3885) projected
  line L862 (54.4744, -9.3885) -> (53.4744, -11.1205) projected
  line L863 (53.4744, -11.1205) -> (51.4744, -11.1205) projected
  line L864 (46.7423, -13.8526) -> (45.7423, -12.1205) projected
  line L865 (45.7423, -12.1205) -> (46.7423, -10.3885) projected
  line L866 (46.7423, -10.3885) -> (48.7423, -10.3885) projected
  line L867 (48.7423, -10.3885) -> (49.7423, -12.1205) projected
  line L868 (49.7423, -12.1205) -> (48.7423, -13.8526) projected
  line L869 (48.7423, -13.8526) -> (46.7423, -13.8526) projected
  line L870 (42.0103, -11.1205) -> (41.0103, -9.3885) projected
  line L871 (41.0103, -9.3885) -> (42.0103, -7.6564) projected
  line L872 (42.0103, -7.6564) -> (44.0103, -7.6564) projected
  line L873 (44.0103, -7.6564) -> (45.0103, -9.3885) projected
  line L874 (45.0103, -9.3885) -> (44.0103, -11.1205) projected
  line L875 (44.0103, -11.1205) -> (42.0103, -11.1205) projected
  line L876 (37.2782, -13.8526) -> (36.2782, -12.1205) projected
  line L877 (36.2782, -12.1205) -> (37.2782, -10.3885) projected
  line L878 (37.2782, -10.3885) -> (39.2782, -10.3885) projected
  line L879 (39.2782, -10.3885) -> (40.2782, -12.1205) projected
  line L880 (40.2782, -12.1205) -> (39.2782, -13.8526) projected
  line L881 (39.2782, -13.8526) -> (37.2782, -13.8526) projected
  line L882 (32.5462, -11.1205) -> (31.5462, -9.3885) projected
  line L883 (31.5462, -9.3885) -> (32.5462, -7.6564) projected
  line L884 (32.5462, -7.6564) -> (34.5462, -7.6564) projected
  line L885 (34.5462, -7.6564) -> (35.5462, -9.3885) projected
  line L886 (35.5462, -9.3885) -> (34.5462, -11.1205) projected
  line L887 (34.5462, -11.1205) -> (32.5462, -11.1205) projected
  line L888 (27.8141, -13.8526) -> (26.8141, -12.1205) projected
  line L889 (26.8141, -12.1205) -> (27.8141, -10.3885) projected
  line L890 (27.8141, -10.3885) -> (29.8141, -10.3885) projected
  line L891 (29.8141, -10.3885) -> (30.8141, -12.1205) projected
  line L892 (30.8141, -12.1205) -> (29.8141, -13.8526) projected
  line L893 (29.8141, -13.8526) -> (27.8141, -13.8526) projected
  line L894 (23.0821, -11.1205) -> (22.0821, -9.3885) projected
  line L895 (22.0821, -9.3885) -> (23.0821, -7.6564) projected
  line L896 (23.0821, -7.6564) -> (25.0821, -7.6564) projected
  line L897 (25.0821, -7.6564) -> (26.0821, -9.3885) projected
  line L898 (26.0821, -9.3885) -> (25.0821, -11.1205) projected
  line L899 (25.0821, -11.1205) -> (23.0821, -11.1205) projected
  line L900 (75.1346, -8.3885) -> (74.1346, -6.6564) projected
  line L901 (74.1346, -6.6564) -> (75.1346, -4.9244) projected
  line L902 (75.1346, -4.9244) -> (77.1346, -4.9244) projected
  line L903 (77.1346, -4.9244) -> (78.1346, -6.6564) projected
  line L904 (78.1346, -6.6564) -> (77.1346, -8.3885) projected
  line L905 (77.1346, -8.3885) -> (75.1346, -8.3885) projected
  line L906 (70.4026, -5.6564) -> (69.4026, -3.9244) projected
  line L907 (69.4026, -3.9244) -> (70.4026, -2.1923) projected
  line L908 (70.4026, -2.1923) -> (72.4026, -2.1923) projected
  line L909 (72.4026, -2.1923) -> (73.4026, -3.9244) projected
  line L910 (73.4026, -3.9244) -> (72.4026, -5.6564) projected
  line L911 (72.4026, -5.6564) -> (70.4026, -5.6564) projected